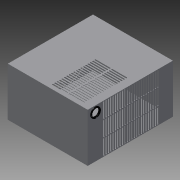
# Autodesk Inventor part: Power Supply
Saved by Autodesk Inventor 2014 SP1 (Build 180222100, 222)
## iProperties
Created: 2014-11-05
Part Number: Power Supply
Material: Generic
Document SubType Name: Modeling
Designer: AlecShufelt
Density: 1 g/cm^3
Appearance: Default
Author: AlecShufelt
Autodesk Inventor part; units mm, degrees
(part 1 of 2)
ref_plane "YZ Plane" through (0, 0, 0) normal (1, 0, 0) x (0, 1, 0)
ref_plane "XZ Plane" through (0, 0, 0) normal (0, 1, 0) x (-1, 0, 0)
ref_plane "XY Plane" through (0, 0, 0) normal (0, 0, 1) x (1, 0, 0)
sketch "Sketch1" plane through (0, 0, 0) normal (0, 1, 0) x (-1, 0, 0)
  line L0 (0, 0) -> (141.224, 0)
  line L1 (141.224, 0) -> (141.224, 150.495)
  line L2 (141.224, 150.495) -> (0, 150.495)
  line L3 (0, 150.495) -> (0, 0)
  dimension "d0" = 141.224
  dimension "d1" = 150.495
  constraints: 8 end point, 2 parallel, 1 horizontal, 1 perpendicular
  measures "d0" distance of L2.end L1.end
  measures "d1" distance of L0.end L1.end
extrude "Extrusion1" add sketch "Sketch1" along normal blind 85.852
sketch "Sketch2" plane through (0, 85.852, 0) normal (0, 1, 0) x (1, 0, 0)
  line L0 (-141.224, 0) -> (-141.224, -150.495) projected
  line L1 (-141.224, -150.495) -> (0, -150.495) projected
  arc A0 (-69.5198, -141.3129) -> (-69.5198, -143.4719) centre (-69.5198, -142.3924) ccw
  line L2 (-69.5198, -143.4719) -> (-44.3738, -143.4719)
  line L3 (-69.5198, -141.3129) -> (-44.3738, -141.3129)
  arc A1 (-44.3738, -143.4719) -> (-44.3738, -141.3129) centre (-44.3738, -142.3924) ccw
  line L4 (-69.5198, -142.3924) -> (-68.4403, -142.3924)
  line L5 (-45.4533, -142.3924) -> (-44.3738, -142.3924)
  line L6 (-69.5198, -139.3317) -> (-44.3738, -139.3317)
  line L7 (-69.5198, -137.1727) -> (-44.3738, -137.1727)
  arc A2 (-44.3738, -139.3317) -> (-44.3738, -137.1727) centre (-44.3738, -138.2522) ccw
  line L8 (-69.5198, -138.2522) -> (-68.4403, -138.2522)
  line L9 (-45.4533, -138.2522) -> (-44.3738, -138.2522)
  arc A3 (-69.5198, -137.1727) -> (-69.5198, -139.3317) centre (-69.5198, -138.2522) ccw
  arc A4 (-69.5198, -133.0325) -> (-69.5198, -135.1915) centre (-69.5198, -134.112) ccw
  line L10 (-69.5198, -135.1915) -> (-44.3738, -135.1915)
  line L11 (-69.5198, -133.0325) -> (-44.3738, -133.0325)
  arc A5 (-44.3738, -135.1915) -> (-44.3738, -133.0325) centre (-44.3738, -134.112) ccw
  line L12 (-69.5198, -134.112) -> (-68.4403, -134.112)
  line L13 (-45.4533, -134.112) -> (-44.3738, -134.112)
  line L14 (-69.5198, -128.8923) -> (-44.3738, -128.8923)
  line L15 (-69.5198, -131.0513) -> (-44.3738, -131.0513)
  line L16 (-69.5198, -129.9718) -> (-68.4403, -129.9718)
  line L17 (-45.4533, -129.9718) -> (-44.3738, -129.9718)
  arc A6 (-44.3738, -131.0513) -> (-44.3738, -128.8923) centre (-44.3738, -129.9718) ccw
  arc A7 (-69.5198, -128.8923) -> (-69.5198, -131.0513) centre (-69.5198, -129.9718) ccw
  line L18 (-69.5198, -124.7521) -> (-44.3738, -124.7521)
  line L19 (-45.4533, -125.8316) -> (-44.3738, -125.8316)
  line L20 (-69.5198, -126.9111) -> (-44.3738, -126.9111)
  arc A8 (-44.3738, -126.9111) -> (-44.3738, -124.7521) centre (-44.3738, -125.8316) ccw
  line L21 (-69.5198, -125.8316) -> (-68.4403, -125.8316)
  arc A9 (-69.5198, -124.7521) -> (-69.5198, -126.9111) centre (-69.5198, -125.8316) ccw
  arc A10 (-69.5198, -120.097) -> (-69.5198, -122.256) centre (-69.5198, -121.1765) ccw
  line L22 (-69.5198, -122.256) -> (-44.3738, -122.256)
  line L23 (-69.5198, -120.097) -> (-44.3738, -120.097)
  arc A11 (-44.3738, -122.256) -> (-44.3738, -120.097) centre (-44.3738, -121.1765) ccw
  line L24 (-69.5198, -121.1765) -> (-68.4403, -121.1765)
  line L25 (-45.4533, -121.1765) -> (-44.3738, -121.1765)
  line L26 (-69.5198, -115.9568) -> (-44.3738, -115.9568)
  line L27 (-69.5198, -118.1158) -> (-44.3738, -118.1158)
  line L28 (-69.5198, -117.0363) -> (-68.4403, -117.0363)
  line L29 (-45.4533, -117.0363) -> (-44.3738, -117.0363)
  arc A12 (-44.3738, -118.1158) -> (-44.3738, -115.9568) centre (-44.3738, -117.0363) ccw
  arc A13 (-69.5198, -115.9568) -> (-69.5198, -118.1158) centre (-69.5198, -117.0363) ccw
  line L30 (-69.5198, -111.8166) -> (-44.3738, -111.8166)
  line L31 (-69.5198, -107.6764) -> (-44.3738, -107.6764)
  line L32 (-45.4533, -108.7559) -> (-44.3738, -108.7559)
  line L33 (-69.5198, -113.9756) -> (-44.3738, -113.9756)
  line L34 (-69.5198, -109.8354) -> (-44.3738, -109.8354)
  arc A14 (-44.3738, -109.8354) -> (-44.3738, -107.6764) centre (-44.3738, -108.7559) ccw
  arc A15 (-44.3738, -113.9756) -> (-44.3738, -111.8166) centre (-44.3738, -112.8961) ccw
  line L35 (-45.4533, -112.8961) -> (-44.3738, -112.8961)
  line L36 (-69.5198, -112.8961) -> (-68.4403, -112.8961)
  line L37 (-69.5198, -108.7559) -> (-68.4403, -108.7559)
  arc A16 (-69.5198, -111.8166) -> (-69.5198, -113.9756) centre (-69.5198, -112.8961) ccw
  arc A17 (-69.5198, -107.6764) -> (-69.5198, -109.8354) centre (-69.5198, -108.7559) ccw
  line L38 (-69.5198, -104.6157) -> (-68.4403, -104.6157)
  line L39 (-69.5198, -103.5362) -> (-44.3738, -103.5362)
  line L40 (-69.5198, -105.6952) -> (-44.3738, -105.6952)
  arc A18 (-69.5198, -103.5362) -> (-69.5198, -105.6952) centre (-69.5198, -104.6157) ccw
  line L41 (-45.4533, -104.6157) -> (-44.3738, -104.6157)
  arc A19 (-44.3738, -105.6952) -> (-44.3738, -103.5362) centre (-44.3738, -104.6157) ccw
  arc A20 (-69.5198, -99.396) -> (-69.5198, -101.555) centre (-69.5198, -100.4755) ccw
  line L42 (-69.5198, -101.555) -> (-44.3738, -101.555)
  line L43 (-69.5198, -99.396) -> (-44.3738, -99.396)
  arc A21 (-44.3738, -101.555) -> (-44.3738, -99.396) centre (-44.3738, -100.4755) ccw
  line L44 (-69.5198, -100.4755) -> (-68.4403, -100.4755)
  line L45 (-45.4533, -100.4755) -> (-44.3738, -100.4755)
  line L46 (-69.5198, -95.2558) -> (-44.3738, -95.2558)
  line L47 (-69.5198, -97.4148) -> (-44.3738, -97.4148)
  line L48 (-69.5198, -96.3353) -> (-68.4403, -96.3353)
  line L49 (-45.4533, -96.3353) -> (-44.3738, -96.3353)
  arc A22 (-44.3738, -97.4148) -> (-44.3738, -95.2558) centre (-44.3738, -96.3353) ccw
  arc A23 (-69.5198, -95.2558) -> (-69.5198, -97.4148) centre (-69.5198, -96.3353) ccw
  line L50 (-69.5198, -91.1156) -> (-44.3738, -91.1156)
  line L51 (-69.5198, -86.9754) -> (-44.3738, -86.9754)
  line L52 (-45.4533, -88.0549) -> (-44.3738, -88.0549)
  line L53 (-69.5198, -93.2746) -> (-44.3738, -93.2746)
  line L54 (-69.5198, -89.1344) -> (-44.3738, -89.1344)
  arc A24 (-44.3738, -89.1344) -> (-44.3738, -86.9754) centre (-44.3738, -88.0549) ccw
  arc A25 (-44.3738, -93.2746) -> (-44.3738, -91.1156) centre (-44.3738, -92.1951) ccw
  line L55 (-45.4533, -92.1951) -> (-44.3738, -92.1951)
  line L56 (-69.5198, -92.1951) -> (-68.4403, -92.1951)
  line L57 (-69.5198, -88.0549) -> (-68.4403, -88.0549)
  arc A26 (-69.5198, -91.1156) -> (-69.5198, -93.2746) centre (-69.5198, -92.1951) ccw
  arc A27 (-69.5198, -86.9754) -> (-69.5198, -89.1344) centre (-69.5198, -88.0549) ccw
  line L58 (-69.5198, -83.9147) -> (-68.4403, -83.9147)
  line L59 (-69.5198, -82.8352) -> (-44.3738, -82.8352)
  line L60 (-69.5198, -84.9942) -> (-44.3738, -84.9942)
  arc A28 (-69.5198, -82.8352) -> (-69.5198, -84.9942) centre (-69.5198, -83.9147) ccw
  line L61 (-45.4533, -83.9147) -> (-44.3738, -83.9147)
  arc A29 (-44.3738, -84.9942) -> (-44.3738, -82.8352) centre (-44.3738, -83.9147) ccw
  arc A30 (-69.5198, -78.695) -> (-69.5198, -80.854) centre (-69.5198, -79.7745) ccw
  line L62 (-69.5198, -80.854) -> (-44.3738, -80.854)
  line L63 (-69.5198, -78.695) -> (-44.3738, -78.695)
  arc A31 (-44.3738, -80.854) -> (-44.3738, -78.695) centre (-44.3738, -79.7745) ccw
  line L64 (-69.5198, -79.7745) -> (-68.4403, -79.7745)
  line L65 (-45.4533, -79.7745) -> (-44.3738, -79.7745)
  line L66 (-69.5198, -74.5548) -> (-44.3738, -74.5548)
  line L67 (-69.5198, -76.7138) -> (-44.3738, -76.7138)
  line L68 (-69.5198, -75.6343) -> (-68.4403, -75.6343)
  line L69 (-45.4533, -75.6343) -> (-44.3738, -75.6343)
  arc A32 (-44.3738, -76.7138) -> (-44.3738, -74.5548) centre (-44.3738, -75.6343) ccw
  arc A33 (-69.5198, -74.5548) -> (-69.5198, -76.7138) centre (-69.5198, -75.6343) ccw
  line L70 (-69.5198, -70.4146) -> (-44.3738, -70.4146)
  line L71 (-69.5198, -66.2744) -> (-44.3738, -66.2744)
  line L72 (-45.4533, -67.3539) -> (-44.3738, -67.3539)
  line L73 (-69.5198, -72.5736) -> (-44.3738, -72.5736)
  line L74 (-69.5198, -68.4334) -> (-44.3738, -68.4334)
  arc A34 (-44.3738, -68.4334) -> (-44.3738, -66.2744) centre (-44.3738, -67.3539) ccw
  arc A35 (-44.3738, -72.5736) -> (-44.3738, -70.4146) centre (-44.3738, -71.4941) ccw
  line L75 (-45.4533, -71.4941) -> (-44.3738, -71.4941)
  line L76 (-69.5198, -71.4941) -> (-68.4403, -71.4941)
  line L77 (-69.5198, -67.3539) -> (-68.4403, -67.3539)
  arc A36 (-69.5198, -70.4146) -> (-69.5198, -72.5736) centre (-69.5198, -71.4941) ccw
  arc A37 (-69.5198, -66.2744) -> (-69.5198, -68.4334) centre (-69.5198, -67.3539) ccw
  arc A38 (-40.0632, -141.3129) -> (-40.0632, -143.4719) centre (-40.0632, -142.3924) ccw
  line L78 (-40.0632, -143.4719) -> (-14.9172, -143.4719)
  line L79 (-40.0632, -141.3129) -> (-14.9172, -141.3129)
  arc A39 (-14.9172, -143.4719) -> (-14.9172, -141.3129) centre (-14.9172, -142.3924) ccw
  line L80 (-40.0632, -142.3924) -> (-38.9837, -142.3924)
  line L81 (-15.9967, -142.3924) -> (-14.9172, -142.3924)
  line L82 (-40.0632, -137.1727) -> (-14.9172, -137.1727)
  line L83 (-40.0632, -139.3317) -> (-14.9172, -139.3317)
  line L84 (-40.0632, -138.2522) -> (-38.9837, -138.2522)
  line L85 (-15.9967, -138.2522) -> (-14.9172, -138.2522)
  arc A40 (-14.9172, -139.3317) -> (-14.9172, -137.1727) centre (-14.9172, -138.2522) ccw
  arc A41 (-40.0632, -137.1727) -> (-40.0632, -139.3317) centre (-40.0632, -138.2522) ccw
  line L86 (-40.0632, -133.0325) -> (-14.9172, -133.0325)
  line L87 (-40.0632, -128.8923) -> (-14.9172, -128.8923)
  line L88 (-15.9967, -129.9718) -> (-14.9172, -129.9718)
  line L89 (-40.0632, -135.1915) -> (-14.9172, -135.1915)
  line L90 (-40.0632, -131.0513) -> (-14.9172, -131.0513)
  arc A42 (-14.9172, -131.0513) -> (-14.9172, -128.8923) centre (-14.9172, -129.9718) ccw
  arc A43 (-14.9172, -135.1915) -> (-14.9172, -133.0325) centre (-14.9172, -134.112) ccw
  line L91 (-15.9967, -134.112) -> (-14.9172, -134.112)
  line L92 (-40.0632, -134.112) -> (-38.9837, -134.112)
  line L93 (-40.0632, -129.9718) -> (-38.9837, -129.9718)
  arc A44 (-40.0632, -133.0325) -> (-40.0632, -135.1915) centre (-40.0632, -134.112) ccw
  arc A45 (-40.0632, -128.8923) -> (-40.0632, -131.0513) centre (-40.0632, -129.9718) ccw
  line L94 (-40.0632, -125.8316) -> (-38.9837, -125.8316)
  line L95 (-40.0632, -124.7521) -> (-14.9172, -124.7521)
  line L96 (-40.0632, -126.9111) -> (-14.9172, -126.9111)
  arc A46 (-40.0632, -124.7521) -> (-40.0632, -126.9111) centre (-40.0632, -125.8316) ccw
  line L97 (-15.9967, -125.8316) -> (-14.9172, -125.8316)
  arc A47 (-14.9172, -126.9111) -> (-14.9172, -124.7521) centre (-14.9172, -125.8316) ccw
  arc A48 (-14.9172, -122.256) -> (-14.9172, -120.097) centre (-14.9172, -121.1765) ccw
  line L98 (-15.9967, -121.1765) -> (-14.9172, -121.1765)
  arc A49 (-14.9172, -118.1158) -> (-14.9172, -115.9568) centre (-14.9172, -117.0363) ccw
  line L99 (-15.9967, -117.0363) -> (-14.9172, -117.0363)
  arc A50 (-14.9172, -113.9756) -> (-14.9172, -111.8166) centre (-14.9172, -112.8961) ccw
  line L100 (-15.9967, -112.8961) -> (-14.9172, -112.8961)
  arc A51 (-14.9172, -109.8354) -> (-14.9172, -107.6764) centre (-14.9172, -108.7559) ccw
  arc A52 (-14.9172, -105.6952) -> (-14.9172, -103.5362) centre (-14.9172, -104.6157) ccw
  line L101 (-15.9967, -104.6157) -> (-14.9172, -104.6157)
  line L102 (-40.0632, -122.256) -> (-14.9172, -122.256)
  line L103 (-40.0632, -120.097) -> (-14.9172, -120.097)
  line L104 (-40.0632, -115.9568) -> (-14.9172, -115.9568)
  line L105 (-40.0632, -118.1158) -> (-14.9172, -118.1158)
  line L106 (-40.0632, -103.5362) -> (-14.9172, -103.5362)
  line L107 (-40.0632, -105.6952) -> (-14.9172, -105.6952)
  line L108 (-40.0632, -113.9756) -> (-14.9172, -113.9756)
  line L109 (-40.0632, -107.6764) -> (-14.9172, -107.6764)
  line L110 (-40.0632, -111.8166) -> (-14.9172, -111.8166)
  line L111 (-40.0632, -109.8354) -> (-14.9172, -109.8354)
  line L112 (-15.9967, -108.7559) -> (-14.9172, -108.7559)
  line L113 (-40.0632, -112.8961) -> (-38.9837, -112.8961)
  arc A53 (-40.0632, -111.8166) -> (-40.0632, -113.9756) centre (-40.0632, -112.8961) ccw
  line L114 (-40.0632, -108.7559) -> (-38.9837, -108.7559)
  arc A54 (-40.0632, -107.6764) -> (-40.0632, -109.8354) centre (-40.0632, -108.7559) ccw
  line L115 (-40.0632, -104.6157) -> (-38.9837, -104.6157)
  arc A55 (-40.0632, -103.5362) -> (-40.0632, -105.6952) centre (-40.0632, -104.6157) ccw
  arc A56 (-40.0632, -120.097) -> (-40.0632, -122.256) centre (-40.0632, -121.1765) ccw
  line L116 (-40.0632, -121.1765) -> (-38.9837, -121.1765)
  line L117 (-40.0632, -117.0363) -> (-38.9837, -117.0363)
  arc A57 (-40.0632, -115.9568) -> (-40.0632, -118.1158) centre (-40.0632, -117.0363) ccw
  arc A58 (-14.9172, -101.555) -> (-14.9172, -99.396) centre (-14.9172, -100.4755) ccw
  line L118 (-15.9967, -100.4755) -> (-14.9172, -100.4755)
  arc A59 (-14.9172, -97.4148) -> (-14.9172, -95.2558) centre (-14.9172, -96.3353) ccw
  line L119 (-15.9967, -96.3353) -> (-14.9172, -96.3353)
  arc A60 (-14.9172, -93.2746) -> (-14.9172, -91.1156) centre (-14.9172, -92.1951) ccw
  line L120 (-15.9967, -92.1951) -> (-14.9172, -92.1951)
  arc A61 (-14.9172, -89.1344) -> (-14.9172, -86.9754) centre (-14.9172, -88.0549) ccw
  arc A62 (-14.9172, -84.9942) -> (-14.9172, -82.8352) centre (-14.9172, -83.9147) ccw
  line L121 (-15.9967, -83.9147) -> (-14.9172, -83.9147)
  line L122 (-40.0632, -101.555) -> (-14.9172, -101.555)
  line L123 (-40.0632, -99.396) -> (-14.9172, -99.396)
  line L124 (-40.0632, -95.2558) -> (-14.9172, -95.2558)
  line L125 (-40.0632, -97.4148) -> (-14.9172, -97.4148)
  line L126 (-40.0632, -82.8352) -> (-14.9172, -82.8352)
  line L127 (-40.0632, -84.9942) -> (-14.9172, -84.9942)
  line L128 (-40.0632, -93.2746) -> (-14.9172, -93.2746)
  line L129 (-40.0632, -86.9754) -> (-14.9172, -86.9754)
  line L130 (-40.0632, -91.1156) -> (-14.9172, -91.1156)
  line L131 (-40.0632, -89.1344) -> (-14.9172, -89.1344)
  line L132 (-15.9967, -88.0549) -> (-14.9172, -88.0549)
  line L133 (-40.0632, -92.1951) -> (-38.9837, -92.1951)
  arc A63 (-40.0632, -91.1156) -> (-40.0632, -93.2746) centre (-40.0632, -92.1951) ccw
  line L134 (-40.0632, -88.0549) -> (-38.9837, -88.0549)
  arc A64 (-40.0632, -86.9754) -> (-40.0632, -89.1344) centre (-40.0632, -88.0549) ccw
  line L135 (-40.0632, -83.9147) -> (-38.9837, -83.9147)
  arc A65 (-40.0632, -82.8352) -> (-40.0632, -84.9942) centre (-40.0632, -83.9147) ccw
  arc A66 (-40.0632, -99.396) -> (-40.0632, -101.555) centre (-40.0632, -100.4755) ccw
  line L136 (-40.0632, -100.4755) -> (-38.9837, -100.4755)
  line L137 (-40.0632, -96.3353) -> (-38.9837, -96.3353)
  arc A67 (-40.0632, -95.2558) -> (-40.0632, -97.4148) centre (-40.0632, -96.3353) ccw
  arc A68 (-14.9172, -80.854) -> (-14.9172, -78.695) centre (-14.9172, -79.7745) ccw
  line L138 (-15.9967, -79.7745) -> (-14.9172, -79.7745)
  arc A69 (-14.9172, -76.7138) -> (-14.9172, -74.5548) centre (-14.9172, -75.6343) ccw
  line L139 (-15.9967, -75.6343) -> (-14.9172, -75.6343)
  arc A70 (-14.9172, -72.5736) -> (-14.9172, -70.4146) centre (-14.9172, -71.4941) ccw
  line L140 (-15.9967, -71.4941) -> (-14.9172, -71.4941)
  arc A71 (-14.9172, -68.4334) -> (-14.9172, -66.2744) centre (-14.9172, -67.3539) ccw
  line L141 (-40.0632, -80.854) -> (-14.9172, -80.854)
  line L142 (-40.0632, -78.695) -> (-14.9172, -78.695)
  line L143 (-40.0632, -74.5548) -> (-14.9172, -74.5548)
  line L144 (-40.0632, -76.7138) -> (-14.9172, -76.7138)
  line L145 (-40.0632, -72.5736) -> (-14.9172, -72.5736)
  line L146 (-40.0632, -66.2744) -> (-14.9172, -66.2744)
  line L147 (-40.0632, -70.4146) -> (-14.9172, -70.4146)
  line L148 (-40.0632, -68.4334) -> (-14.9172, -68.4334)
  line L149 (-15.9967, -67.3539) -> (-14.9172, -67.3539)
  line L150 (-40.0632, -71.4941) -> (-38.9837, -71.4941)
  arc A72 (-40.0632, -70.4146) -> (-40.0632, -72.5736) centre (-40.0632, -71.4941) ccw
  line L151 (-40.0632, -67.3539) -> (-38.9837, -67.3539)
  arc A73 (-40.0632, -66.2744) -> (-40.0632, -68.4334) centre (-40.0632, -67.3539) ccw
  arc A74 (-40.0632, -78.695) -> (-40.0632, -80.854) centre (-40.0632, -79.7745) ccw
  line L152 (-40.0632, -79.7745) -> (-38.9837, -79.7745)
  line L153 (-40.0632, -75.6343) -> (-38.9837, -75.6343)
  arc A75 (-40.0632, -74.5548) -> (-40.0632, -76.7138) centre (-40.0632, -75.6343) ccw
  dimension "d4" = 2.159
  dimension "d5" = 25.146
  dimension "d6" = 71.7042
  dimension "d7" = 8.1026
  dimension "d8" = 25.146
  dimension "d9" = 4.1402
  dimension "d10" = 2.159
  dimension "d11" = 25.146
  dimension "d12" = 25.146
  dimension "d13" = 4.1402
  dimension "d14" = 4.1402
  dimension "d15" = 25.146
  dimension "d16" = 4.1402
  dimension "d17" = 2.159
  dimension "d18" = 25.146
  dimension "d19" = 25.146
  dimension "d20" = 4.1402
  dimension "d21" = 2.159
  dimension "d22" = 25.146
  dimension "d23" = 25.146
  dimension "d24" = 4.1402
  dimension "d25" = 4.1402
  dimension "d26" = 25.146
  dimension "d27" = 4.1402
  dimension "d28" = 2.159
  dimension "d29" = 25.146
  dimension "d30" = 25.146
  dimension "d31" = 4.1402
  dimension "d32" = 2.159
  dimension "d33" = 25.146
  dimension "d34" = 25.146
  dimension "d35" = 4.1402
  dimension "d36" = 4.1402
  dimension "d37" = 25.146
  dimension "d38" = 4.1402
  dimension "d39" = 2.159
  dimension "d40" = 25.146
  dimension "d41" = 25.146
  dimension "d42" = 4.1402
  dimension "d43" = 2.159
  dimension "d44" = 25.146
  dimension "d45" = 25.146
  dimension "d46" = 4.1402
  dimension "d47" = 4.1402
  dimension "d50" = 4.1402
  dimension "d51" = 4.1402
  dimension "d52" = 2.159
  dimension "d53" = 25.146
  dimension "d54" = 25.146
  dimension "d55" = 4.1402
  dimension "d56" = 2.159
  dimension "d57" = 25.146
  dimension "d58" = 25.146
  dimension "d59" = 4.1402
  dimension "d60" = 4.1402
  dimension "d61" = 25.146
  dimension "d62" = 4.1402
  dimension "d63" = 2.159
  dimension "d64" = 25.146
  dimension "d65" = 25.146
  dimension "d66" = 4.1402
  dimension "d67" = 2.159
  dimension "d68" = 25.146
  dimension "d69" = 25.146
  constraints: 304 end point, 152 point on circle, 114 parallel, 76 centre point, 60 coincident, 32 tangent
  measures "d4" diameter of A0
  measures "d5" distance of L4.start L5.end
  measures "d6" distance from line of L0 L4.start
  measures "d7" distance from line of L1 L4.start
  measures "d8" distance of L8.start L9.end
  measures "d9" distance between parallel lines of L9 L5
  measures "d10" diameter of A4
  measures "d11" distance of L12.start L13.end
  measures "d12" distance of L16.start L17.end
  measures "d13" distance between parallel lines of L17 L13
  measures "d14" distance of L9.end L13.end
  measures "d15" distance of L21.start L19.end
  measures "d16" distance of L17.end L19.end
  measures "d17" diameter of A10
  measures "d18" distance of L24.start L25.end
  measures "d19" distance of L28.start L29.end
  measures "d20" distance between parallel lines of L29 L25
  measures "d21" diameter of A16
  measures "d22" distance of L36.start L35.end
  measures "d23" distance of L37.start L32.end
  measures "d24" distance between parallel lines of L32 L35
  measures "d25" distance of L29.end L35.end
  measures "d26" distance of L38.start L41.end
  measures "d27" distance of L32.end L41.end
  measures "d28" diameter of A20
  measures "d29" distance of L44.start L45.end
  measures "d30" distance of L48.start L49.end
  measures "d31" distance between parallel lines of L49 L45
  measures "d32" diameter of A26
  measures "d33" distance of L56.start L55.end
  measures "d34" distance of L57.start L52.end
  measures "d35" distance between parallel lines of L52 L55
  measures "d36" distance of L49.end L55.end
  measures "d37" distance of L58.start L61.end
  measures "d38" distance of L52.end L61.end
  measures "d39" diameter of A30
  measures "d40" distance of L64.start L65.end
  measures "d41" distance of L68.start L69.end
  measures "d42" distance between parallel lines of L69 L65
  measures "d43" diameter of A36
  measures "d44" distance of L76.start L75.end
  measures "d45" distance of L77.start L72.end
  measures "d46" distance between parallel lines of L72 L75
  measures "d47" distance of L69.end L75.end
  measures "d50" distance of A21.centre L41.end
  measures "d51" distance of L61.end A31.centre
  measures "d52" diameter of A38
  measures "d53" distance of L80.start L81.end
  measures "d54" distance of L84.start L85.end
  measures "d55" distance between parallel lines of L85 L81
  measures "d56" diameter of A44
  measures "d57" distance of L92.start L91.end
  measures "d58" distance of L93.start L88.end
  measures "d59" distance between parallel lines of L88 L91
  measures "d60" distance of L85.end L91.end
  measures "d61" distance of L94.start L97.end
  measures "d62" distance of L88.end L97.end
  measures "d63" diameter of A56
  measures "d64" distance of L116.start L98.end
  measures "d65" distance of L117.start L99.end
  measures "d66" distance between parallel lines of L99 L98
  measures "d67" diameter of A53
  measures "d68" distance of L113.start L100.end
  measures "d69" distance of L114.start L112.end
extrude "Extrusion2" cut sketch "Sketch2" against normal blind 508
sketch "Sketch4" plane through (0, 0, 0) normal (0, -1, 0) x (1, 0, 0)
  line L0 (-40.0632, 72.5736) -> (-14.9172, 72.5736) projected
  arc A0 (-14.9172, 70.4146) -> (-14.9172, 72.5736) centre (-14.9172, 71.4941) ccw projected
  line L1 (-14.9172, 70.4146) -> (-40.0632, 70.4146) projected
  arc A1 (-40.0632, 72.5736) -> (-40.0632, 70.4146) centre (-40.0632, 71.4941) ccw projected
  line L2 (-40.0632, 80.854) -> (-14.9172, 80.854) projected
  arc A2 (-14.9172, 78.695) -> (-14.9172, 80.854) centre (-14.9172, 79.7745) ccw projected
  line L3 (-14.9172, 78.695) -> (-40.0632, 78.695) projected
  arc A3 (-40.0632, 80.854) -> (-40.0632, 78.695) centre (-40.0632, 79.7745) ccw projected
  arc A4 (-14.9172, 86.9754) -> (-14.9172, 89.1344) centre (-14.9172, 88.0549) ccw projected
  line L4 (-14.9172, 86.9754) -> (-40.0632, 86.9754) projected
  arc A5 (-40.0632, 89.1344) -> (-40.0632, 86.9754) centre (-40.0632, 88.0549) ccw projected
  line L5 (-40.0632, 89.1344) -> (-14.9172, 89.1344) projected
  arc A6 (-40.0632, 97.4148) -> (-40.0632, 95.2558) centre (-40.0632, 96.3353) ccw projected
  line L6 (-40.0632, 97.4148) -> (-14.9172, 97.4148) projected
  arc A7 (-14.9172, 95.2558) -> (-14.9172, 97.4148) centre (-14.9172, 96.3353) ccw projected
  line L7 (-14.9172, 95.2558) -> (-40.0632, 95.2558) projected
  line L8 (-40.0632, 113.9756) -> (-14.9172, 113.9756) projected
  arc A8 (-14.9172, 111.8166) -> (-14.9172, 113.9756) centre (-14.9172, 112.8961) ccw projected
  line L9 (-14.9172, 111.8166) -> (-40.0632, 111.8166) projected
  arc A9 (-40.0632, 113.9756) -> (-40.0632, 111.8166) centre (-40.0632, 112.8961) ccw projected
  arc A10 (-14.9172, 103.5362) -> (-14.9172, 105.6952) centre (-14.9172, 104.6157) ccw projected
  line L10 (-14.9172, 103.5362) -> (-40.0632, 103.5362) projected
  arc A11 (-40.0632, 105.6952) -> (-40.0632, 103.5362) centre (-40.0632, 104.6157) ccw projected
  line L11 (-40.0632, 105.6952) -> (-14.9172, 105.6952) projected
  arc A12 (-40.0632, 131.0513) -> (-40.0632, 128.8923) centre (-40.0632, 129.9718) ccw projected
  line L12 (-40.0632, 131.0513) -> (-14.9172, 131.0513) projected
  arc A13 (-14.9172, 128.8923) -> (-14.9172, 131.0513) centre (-14.9172, 129.9718) ccw projected
  line L13 (-14.9172, 128.8923) -> (-40.0632, 128.8923) projected
  arc A14 (-40.0632, 139.3317) -> (-40.0632, 137.1727) centre (-40.0632, 138.2522) ccw projected
  line L14 (-40.0632, 139.3317) -> (-14.9172, 139.3317) projected
  arc A15 (-14.9172, 137.1727) -> (-14.9172, 139.3317) centre (-14.9172, 138.2522) ccw projected
  line L15 (-14.9172, 137.1727) -> (-40.0632, 137.1727) projected
  arc A16 (-40.0632, 126.9111) -> (-40.0632, 124.7521) centre (-40.0632, 125.8316) ccw projected
  line L16 (-40.0632, 126.9111) -> (-14.9172, 126.9111) projected
  arc A17 (-14.9172, 124.7521) -> (-14.9172, 126.9111) centre (-14.9172, 125.8316) ccw projected
  line L17 (-14.9172, 124.7521) -> (-40.0632, 124.7521) projected
  arc A18 (-44.3738, 66.2744) -> (-44.3738, 68.4334) centre (-44.3738, 67.3539) ccw projected
  line L18 (-44.3738, 66.2744) -> (-69.5198, 66.2744) projected
  arc A19 (-69.5198, 68.4334) -> (-69.5198, 66.2744) centre (-69.5198, 67.3539) ccw projected
  line L19 (-69.5198, 68.4334) -> (-44.3738, 68.4334) projected
  arc A20 (-44.3738, 74.5548) -> (-44.3738, 76.7138) centre (-44.3738, 75.6343) ccw projected
  line L20 (-44.3738, 74.5548) -> (-69.5198, 74.5548) projected
  arc A21 (-69.5198, 76.7138) -> (-69.5198, 74.5548) centre (-69.5198, 75.6343) ccw projected
  line L21 (-69.5198, 76.7138) -> (-44.3738, 76.7138) projected
  arc A22 (-44.3738, 82.8352) -> (-44.3738, 84.9942) centre (-44.3738, 83.9147) ccw projected
  line L22 (-44.3738, 82.8352) -> (-69.5198, 82.8352) projected
  arc A23 (-69.5198, 84.9942) -> (-69.5198, 82.8352) centre (-69.5198, 83.9147) ccw projected
  line L23 (-69.5198, 84.9942) -> (-44.3738, 84.9942) projected
  arc A24 (-44.3738, 91.1156) -> (-44.3738, 93.2746) centre (-44.3738, 92.1951) ccw projected
  line L24 (-44.3738, 91.1156) -> (-69.5198, 91.1156) projected
  arc A25 (-69.5198, 93.2746) -> (-69.5198, 91.1156) centre (-69.5198, 92.1951) ccw projected
  line L25 (-69.5198, 93.2746) -> (-44.3738, 93.2746) projected
  arc A26 (-44.3738, 99.396) -> (-44.3738, 101.555) centre (-44.3738, 100.4755) ccw projected
  line L26 (-44.3738, 99.396) -> (-69.5198, 99.396) projected
  arc A27 (-69.5198, 101.555) -> (-69.5198, 99.396) centre (-69.5198, 100.4755) ccw projected
  line L27 (-69.5198, 101.555) -> (-44.3738, 101.555) projected
  arc A28 (-44.3738, 107.6764) -> (-44.3738, 109.8354) centre (-44.3738, 108.7559) ccw projected
  line L28 (-44.3738, 107.6764) -> (-69.5198, 107.6764) projected
  arc A29 (-69.5198, 109.8354) -> (-69.5198, 107.6764) centre (-69.5198, 108.7559) ccw projected
  line L29 (-69.5198, 109.8354) -> (-44.3738, 109.8354) projected
  arc A30 (-44.3738, 115.9568) -> (-44.3738, 118.1158) centre (-44.3738, 117.0363) ccw projected
  line L30 (-44.3738, 115.9568) -> (-69.5198, 115.9568) projected
  arc A31 (-69.5198, 118.1158) -> (-69.5198, 115.9568) centre (-69.5198, 117.0363) ccw projected
  line L31 (-69.5198, 118.1158) -> (-44.3738, 118.1158) projected
  arc A32 (-69.5198, 126.9111) -> (-69.5198, 124.7521) centre (-69.5198, 125.8316) ccw projected
  line L32 (-69.5198, 126.9111) -> (-44.3738, 126.9111) projected
  arc A33 (-44.3738, 124.7521) -> (-44.3738, 126.9111) centre (-44.3738, 125.8316) ccw projected
  line L33 (-44.3738, 124.7521) -> (-69.5198, 124.7521) projected
  line L34 (-69.5198, 135.1915) -> (-44.3738, 135.1915) projected
  arc A34 (-44.3738, 133.0325) -> (-44.3738, 135.1915) centre (-44.3738, 134.112) ccw projected
  line L35 (-44.3738, 133.0325) -> (-69.5198, 133.0325) projected
  arc A35 (-69.5198, 135.1915) -> (-69.5198, 133.0325) centre (-69.5198, 134.112) ccw projected
  arc A36 (-44.3738, 141.3129) -> (-44.3738, 143.4719) centre (-44.3738, 142.3924) ccw projected
  line L36 (-44.3738, 141.3129) -> (-69.5198, 141.3129) projected
  arc A37 (-69.5198, 143.4719) -> (-69.5198, 141.3129) centre (-69.5198, 142.3924) ccw projected
  line L37 (-69.5198, 143.4719) -> (-44.3738, 143.4719) projected
  arc A38 (-69.5198, 139.3317) -> (-69.5198, 137.1727) centre (-69.5198, 138.2522) ccw projected
  line L38 (-69.5198, 139.3317) -> (-44.3738, 139.3317) projected
  arc A39 (-44.3738, 137.1727) -> (-44.3738, 139.3317) centre (-44.3738, 138.2522) ccw projected
  line L39 (-44.3738, 137.1727) -> (-69.5198, 137.1727) projected
  line L40 (-44.3738, 128.8923) -> (-69.5198, 128.8923) projected
  arc A40 (-69.5198, 131.0513) -> (-69.5198, 128.8923) centre (-69.5198, 129.9718) ccw projected
  line L41 (-69.5198, 131.0513) -> (-44.3738, 131.0513) projected
  arc A41 (-44.3738, 128.8923) -> (-44.3738, 131.0513) centre (-44.3738, 129.9718) ccw projected
  arc A42 (-44.3738, 120.097) -> (-44.3738, 122.256) centre (-44.3738, 121.1765) ccw projected
  line L42 (-44.3738, 120.097) -> (-69.5198, 120.097) projected
  arc A43 (-69.5198, 122.256) -> (-69.5198, 120.097) centre (-69.5198, 121.1765) ccw projected
  line L43 (-69.5198, 122.256) -> (-44.3738, 122.256) projected
  arc A44 (-44.3738, 111.8166) -> (-44.3738, 113.9756) centre (-44.3738, 112.8961) ccw projected
  line L44 (-44.3738, 111.8166) -> (-69.5198, 111.8166) projected
  arc A45 (-69.5198, 113.9756) -> (-69.5198, 111.8166) centre (-69.5198, 112.8961) ccw projected
  line L45 (-69.5198, 113.9756) -> (-44.3738, 113.9756) projected
  arc A46 (-44.3738, 103.5362) -> (-44.3738, 105.6952) centre (-44.3738, 104.6157) ccw projected
  line L46 (-44.3738, 103.5362) -> (-69.5198, 103.5362) projected
  arc A47 (-69.5198, 105.6952) -> (-69.5198, 103.5362) centre (-69.5198, 104.6157) ccw projected
  line L47 (-69.5198, 105.6952) -> (-44.3738, 105.6952) projected
  arc A48 (-44.3738, 95.2558) -> (-44.3738, 97.4148) centre (-44.3738, 96.3353) ccw projected
  line L48 (-44.3738, 95.2558) -> (-69.5198, 95.2558) projected
  arc A49 (-69.5198, 97.4148) -> (-69.5198, 95.2558) centre (-69.5198, 96.3353) ccw projected
  line L49 (-69.5198, 97.4148) -> (-44.3738, 97.4148) projected
  arc A50 (-44.3738, 86.9754) -> (-44.3738, 89.1344) centre (-44.3738, 88.0549) ccw projected
  line L50 (-44.3738, 86.9754) -> (-69.5198, 86.9754) projected
  arc A51 (-69.5198, 89.1344) -> (-69.5198, 86.9754) centre (-69.5198, 88.0549) ccw projected
  line L51 (-69.5198, 89.1344) -> (-44.3738, 89.1344) projected
  arc A52 (-44.3738, 78.695) -> (-44.3738, 80.854) centre (-44.3738, 79.7745) ccw projected
  line L52 (-44.3738, 78.695) -> (-69.5198, 78.695) projected
  arc A53 (-69.5198, 80.854) -> (-69.5198, 78.695) centre (-69.5198, 79.7745) ccw projected
  line L53 (-69.5198, 80.854) -> (-44.3738, 80.854) projected
  arc A54 (-44.3738, 70.4146) -> (-44.3738, 72.5736) centre (-44.3738, 71.4941) ccw projected
  line L54 (-44.3738, 70.4146) -> (-69.5198, 70.4146) projected
  arc A55 (-69.5198, 72.5736) -> (-69.5198, 70.4146) centre (-69.5198, 71.4941) ccw projected
  line L55 (-69.5198, 72.5736) -> (-44.3738, 72.5736) projected
  line L56 (-40.0632, 122.256) -> (-14.9172, 122.256) projected
  arc A56 (-14.9172, 120.097) -> (-14.9172, 122.256) centre (-14.9172, 121.1765) ccw projected
  line L57 (-14.9172, 120.097) -> (-40.0632, 120.097) projected
  arc A57 (-40.0632, 122.256) -> (-40.0632, 120.097) centre (-40.0632, 121.1765) ccw projected
  line L58 (-40.0632, 143.4719) -> (-14.9172, 143.4719) projected
  arc A58 (-14.9172, 141.3129) -> (-14.9172, 143.4719) centre (-14.9172, 142.3924) ccw projected
  line L59 (-14.9172, 141.3129) -> (-40.0632, 141.3129) projected
  arc A59 (-40.0632, 143.4719) -> (-40.0632, 141.3129) centre (-40.0632, 142.3924) ccw projected
  line L60 (-40.0632, 135.1915) -> (-14.9172, 135.1915) projected
  arc A60 (-14.9172, 133.0325) -> (-14.9172, 135.1915) centre (-14.9172, 134.112) ccw projected
  line L61 (-14.9172, 133.0325) -> (-40.0632, 133.0325) projected
  arc A61 (-40.0632, 135.1915) -> (-40.0632, 133.0325) centre (-40.0632, 134.112) ccw projected
  arc A62 (-14.9172, 107.6764) -> (-14.9172, 109.8354) centre (-14.9172, 108.7559) ccw projected
  line L62 (-14.9172, 107.6764) -> (-40.0632, 107.6764) projected
  arc A63 (-40.0632, 109.8354) -> (-40.0632, 107.6764) centre (-40.0632, 108.7559) ccw projected
  line L63 (-40.0632, 109.8354) -> (-14.9172, 109.8354) projected
  arc A64 (-14.9172, 99.396) -> (-14.9172, 101.555) centre (-14.9172, 100.4755) ccw projected
  line L64 (-14.9172, 99.396) -> (-40.0632, 99.396) projected
  arc A65 (-40.0632, 101.555) -> (-40.0632, 99.396) centre (-40.0632, 100.4755) ccw projected
  line L65 (-40.0632, 101.555) -> (-14.9172, 101.555) projected
  arc A66 (-40.0632, 118.1158) -> (-40.0632, 115.9568) centre (-40.0632, 117.0363) ccw projected
  line L66 (-40.0632, 118.1158) -> (-14.9172, 118.1158) projected
  arc A67 (-14.9172, 115.9568) -> (-14.9172, 118.1158) centre (-14.9172, 117.0363) ccw projected
  line L67 (-14.9172, 115.9568) -> (-40.0632, 115.9568) projected
  arc A68 (-14.9172, 91.1156) -> (-14.9172, 93.2746) centre (-14.9172, 92.1951) ccw projected
  line L68 (-14.9172, 91.1156) -> (-40.0632, 91.1156) projected
  arc A69 (-40.0632, 93.2746) -> (-40.0632, 91.1156) centre (-40.0632, 92.1951) ccw projected
  line L69 (-40.0632, 93.2746) -> (-14.9172, 93.2746) projected
  line L70 (-40.0632, 84.9942) -> (-14.9172, 84.9942) projected
  arc A70 (-14.9172, 82.8352) -> (-14.9172, 84.9942) centre (-14.9172, 83.9147) ccw projected
  line L71 (-14.9172, 82.8352) -> (-40.0632, 82.8352) projected
  arc A71 (-40.0632, 84.9942) -> (-40.0632, 82.8352) centre (-40.0632, 83.9147) ccw projected
  line L72 (-40.0632, 76.7138) -> (-14.9172, 76.7138) projected
  arc A72 (-14.9172, 74.5548) -> (-14.9172, 76.7138) centre (-14.9172, 75.6343) ccw projected
  line L73 (-14.9172, 74.5548) -> (-40.0632, 74.5548) projected
  arc A73 (-40.0632, 76.7138) -> (-40.0632, 74.5548) centre (-40.0632, 75.6343) ccw projected
  line L74 (-40.0632, 68.4334) -> (-14.9172, 68.4334) projected
  arc A74 (-14.9172, 66.2744) -> (-14.9172, 68.4334) centre (-14.9172, 67.3539) ccw projected
  line L75 (-14.9172, 66.2744) -> (-40.0632, 66.2744) projected
  arc A75 (-40.0632, 68.4334) -> (-40.0632, 66.2744) centre (-40.0632, 67.3539) ccw projected
  line L76 (-141.224, 150.495) -> (0, 150.495) projected
  line L77 (-141.224, 0) -> (-141.224, 150.495) projected
  line L78 (-140.1318, 149.4028) -> (-1.0922, 149.4028)
  line L79 (-1.0922, 149.4028) -> (-1.0922, 1.0922)
  line L80 (-1.0922, 1.0922) -> (-140.1318, 1.0922)
  line L81 (-140.1318, 1.0922) -> (-140.1318, 149.4028)
  dimension "d102" = 139.0396
  dimension "d103" = 148.3106
  dimension "d104" = 1.0922
  dimension "d105" = 1.0922
  constraints: 8 end point, 2 parallel, 1 horizontal, 1 perpendicular
  measures "d102" distance of L79.end L80.end
  measures "d103" distance of L78.end L79.end
  measures "d104" distance between parallel lines of L76 L78
  measures "d105" distance between parallel lines of L77 L81
extrude "Extrusion3" cut sketch "Sketch4" against normal blind 85.09
sketch "Sketch5" plane through (0, 0, 0) normal (0, -1, 0) x (1, 0, 0)
  line L0 (-140.1318, 1.0922) -> (-140.1318, 149.4028) projected
  line L1 (-140.1318, 149.4028) -> (-1.0922, 149.4028) projected
  line L2 (-1.0922, 149.4028) -> (-1.0922, 1.0922) projected
  line L3 (-1.0922, 1.0922) -> (-140.1318, 1.0922) projected
  line L4 (-141.224, 150.495) -> (0, 150.495)
  line L5 (0, 150.495) -> (0, 0)
  line L6 (0, 0) -> (-141.224, 0)
  line L7 (-141.224, 0) -> (-141.224, 150.495)
  constraints: 8 end point, 2 parallel, 1 horizontal, 1 perpendicular
extrude "Extrusion4" add sketch "Sketch5" against normal blind 1.0922 contours L0 L1 L2 L3